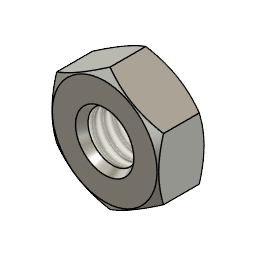
Mounting Plate (Autodesk Fusion 360 archive; units mm, degrees)
design "Hexagon Regular Nut ISO 4032 - M3 Steel 6 Plain"
description: Hexagon Regular Nut ISO 4032 - M3
part number: ISO 4032 - M3 Steel 6 Plain
Autodesk Fusion 360 part; units mm, degrees
sketch "Sketch1" plane through (0, 0, 0) normal (0, 1, 0) x (1, 0, 0)
  line L0 (0, 0) -> (0, -2.4)
  line L1 (-1.5, 0) -> (-2.695, 0)
  line L2 (-2.695, 0) -> (-3.1763, -0.2778)
  line L3 (-3.1763, -0.2778) -> (-3.1763, -2.1222)
  line L4 (-3.1763, -2.1222) -> (-2.695, -2.4)
  line L5 (-2.695, -2.4) -> (-1.5, -2.4)
  line L6 (-1.5, -2.4) -> (-1.5, 0)
  dimension "d121" = 3
  dimension "d122" = 30
  dimension "d123" = 30
  dimension "d128" = 6.3525
  dimension "d172" = 5.39
  dimension "d179" = 2.4
  constraint vertical L0
  constraint coincident L0 L0.end
  constraint coincident origin L0
  constraint horizontal L1
  constraint coincident L0.start L1
  constraint coincident L0.start origin
  constraint coincident L0.end L5
  constraint vertical L1.end L4.end
  measures "d122" angle of L1 L2
  measures "d123" angle of L4 L5
  measures "d179" distance of L1 L5
revolve "Revolve1" add sketch "Sketch1" angle 360 about axis through (0, 0, 0) along (0, 0, 1)
sketch "Sketch8" plane through (0, 0, 2.4) normal (0, 0, 1) x (1, 0, 0)
  line L0 (-2.75, -1.5894) -> (-2.75, 1.5894)
  circle A0 centre (0, 0) radius 1.5
  circle A1 centre (0, 0) radius 3.1763
  dimension "d114" = 2.75
  constraint coincident L0.end A1
  constraint coincident L0.start A1
  constraint vertical L0
  measures "d114" distance of A0.centre L0
extrude "Extrude5" cut sketch "Sketch8" against normal blind 2.4 contours L0 A1 picked at (-2.8188, -0.3871)
pattern_circular "C-Pattern2" count 6 over 360 about axis through (0, 0, 1.75) along (0, 0, 1) of "Extrude5"
thread "Thread3" "ISO Metric profile 3.0 M3x0.5 M3x0.5 6H" major diameter 3.086 minor diameter 2.529 pitch 0.5 angle 60 resizes the face on face at (-1.4925, 0.1494, 1.6)
sketch "Sketch12" plane through (0, 0, 0) normal (0, 1, 0) x (1, 0, 0)
  line L0 (-1.5, 0) -> (0, 0)
  line L1 (-0.8072, -1.2) -> (-1.5, 0)
  line L2 (-1.5, -2.4) -> (0, -2.4)
  line L3 (-0.8072, -1.2) -> (-1.5, -2.4)
  line L4 (0, 0) -> (0, -2.4)
  dimension "d169" = 60
  dimension "d177" = 1.5
  dimension "d178" = 60
  constraint horizontal L0
  constraint coincident L1.start L3.start
  constraint vertical L0.start L2.start
  constraint coincident L2.end L4.end
  constraint coincident L0.end L4.start
  constraint perpendicular L2 L4
  measures "d169" angle of L2 L3
  measures "d177" distance of L0.start L4
  measures "d178" angle of L0 L1
revolve "Revolve3" cut sketch "Sketch12" angle 360 about axis through (0, 0, 1.75) along (0, 0, 1)
equation "adsk_nheig = 2.40 mm"
equation "adsk_maxdia = 6.3525 mm"
equation "adsk_nomdia = 3.00 mm"
equation "d89 = -adsk_nheig"
equation "adsk_waflat = 5.50 mm"
equation "d114 = adsk_waflat / 2"
equation "adsk_chamang1 = 30.00 deg"
equation "adsk_chamang2 = 30.00 deg"
equation "d121 = adsk_nomdia"
equation "d122 = adsk_chamang1"
equation "d123 = adsk_chamang2"
equation "d128 = adsk_maxdia"
equation "d163 = adsk_nheig"
equation "adsk_beardia = 5.39 mm"
equation "d172 = adsk_beardia"
equation "d177 = adsk_nomdia * 0.5"
equation "d179 = adsk_nheig"

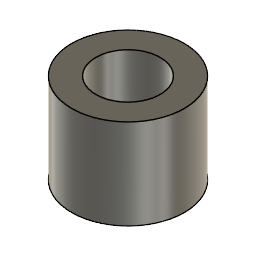
design "Standoff"
part number: 2026-01-10-15-52-55-500
Autodesk Fusion 360 part; units mm, degrees
sketch "Base" plane through (0, 0, 0) normal (0, 0, 1) x (1, 0, 0)
  circle A0 centre (0, 0) radius 5
  circle A1 centre (0, 0) radius 2.85
  circle A2 centre (0, 0) radius 2.2
  dimension "d1" = 10
  dimension "d2" = 5.7
  dimension "d3" = 4.4
  constraint coincident A0.centre A1.centre
  constraint concentric A1 A2
  measures "d1" diameter of A0
  measures "d2" diameter of A1
  measures "d3" diameter of A2
extrude "Extrude1" add sketch "Base" along normal blind 8 contours A0
extrude "Extrude2" add sketch "Base" along normal blind 2 contours A1
equation "d1 = outer_diameter"
equation "d2 = 0.95 * insert_diameter"
equation "d3 = 1.1 * inner_diameter"
equation "d4 = height"
equation "d6 = height - insert_height"
equation "outer_diameter = 10 mm"
equation "inner_diameter = 4 mm"
equation "insert_diameter = 6 mm"
equation "insert_height = 6 mm"
equation "height = 8 mm"

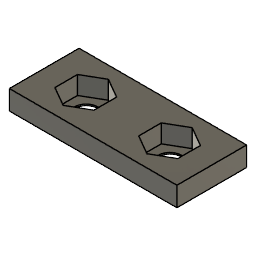
design "Bottom Connector"
part number: 2026-01-10-16-39-12-979
Autodesk Fusion 360 part; units mm, degrees
sketch "Base" plane through (0, 0, 0) normal (0, 0, 1) x (1, 0, 0)
  line L0 (12, 5) -> (-12, 5)
  line L1 (-12, 5) -> (-12, -5)
  line L2 (-12, -5) -> (12, -5)
  line L3 (12, -5) -> (12, 5)
  line L4 (12, 5) -> (-12, -5) construction
  line L5 (-12, 5) -> (12, -5) construction
  circle A0 centre (6, 0) radius 1.65
  circle A1 centre (-6, 0) radius 1.65
  dimension "d110" = 24
  dimension "d111" = 10
  dimension "d112" = 3.3
  dimension "d113" = 3.3
  constraint horizontal L0
  constraint perpendicular L0 L1
  constraint parallel L0 L2
  constraint parallel L1 L3
  constraint coincident L4 origin
  constraint coincident L5 origin
  measures "d110" distance of L1.end L2.end
  measures "d111" distance of L0.end L1.end
  measures "d112" diameter of A0
  measures "d113" diameter of A1
extrude "Extrude27" add sketch "Base" along normal blind 0.5
sketch "Nut Holders" plane through (0, 0, 0) normal (0, 0, 1) x (1, 0, 0)
  line L0 (-12, 5, 0.5) -> (12, 5, 0.5)
  line L1 (12, 5, 0.5) -> (12, -5, 0.5)
  line L2 (12, -5, 0.5) -> (-12, -5, 0.5)
  line L3 (-12, -5, 0.5) -> (-12, 5, 0.5)
  line L4 (-3.25, 1.6166, 0.5) -> (-6.05, 3.2332, 0.5)
  line L5 (-6.05, 3.2332, 0.5) -> (-8.85, 1.6166, 0.5)
  line L6 (-8.85, 1.6166, 0.5) -> (-8.85, -1.6166, 0.5)
  line L7 (-8.85, -1.6166, 0.5) -> (-6.05, -3.2332, 0.5)
  line L8 (-6.05, -3.2332, 0.5) -> (-3.25, -1.6166, 0.5)
  line L9 (-3.25, -1.6166, 0.5) -> (-3.25, 1.6166, 0.5)
  line L10 (8.75, 1.6166, 0.5) -> (5.95, 3.2332, 0.5)
  line L11 (5.95, 3.2332, 0.5) -> (3.15, 1.6166, 0.5)
  line L12 (3.15, 1.6166, 0.5) -> (3.15, -1.6166, 0.5)
  line L13 (3.15, -1.6166, 0.5) -> (5.95, -3.2332, 0.5)
  line L14 (5.95, -3.2332, 0.5) -> (8.75, -1.6166, 0.5)
  line L15 (8.75, -1.6166, 0.5) -> (8.75, 1.6166, 0.5)
  point P0 (-6.05, 0)
  point P1 (5.95, 0)
  dimension "d116" = 2.8
  dimension "d117" = 2.8
extrude "Extrude28" add sketch "Nut Holders" along normal blind 2.5 contours L0 L1 L2 L3 in plane through (0, 0, 0.5) normal (0, 0, 1)
extrude "Extrude29" cut 1 faces at (-8.45, 0, 0.5) along direction (0, 0, -1) blind 0.1
extrude "Extrude30" cut 1 faces at (3.55, 0, 0.5) along direction (0, 0, -1) blind 0.1
extrude "Extrude31" cut 1 faces at (-10.55, 0, 0) along direction (0, 0, 1) blind 0.2
move_body "Move12" bodies 1 to x (1, 0, 0) y (0, 1, 0) z (0, 0, 1) at (0, 0, -0.2)
named bodies: "Body1"

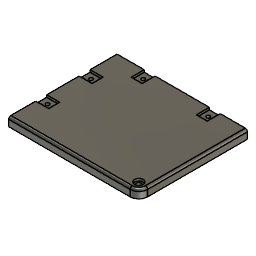
design "Corner"
part number: 2026-01-10-21-06-03-515
Autodesk Fusion 360 part; units mm, degrees
sketch "Base" plane through (0, 0, 0) normal (0, 0, 1) x (1, 0, 0)
  line L0 (60, 50) -> (-60, 50)
  line L1 (-60, 50) -> (-60, -50)
  line L2 (-60, -50) -> (60, -50)
  line L3 (60, -50) -> (60, 50)
  line L4 (60, 50) -> (-60, -50) construction
  line L5 (-60, 50) -> (60, -50) construction
  dimension "d48" = 120
  dimension "d49" = 100
  constraint horizontal L0
  constraint perpendicular L0 L1
  constraint parallel L0 L2
  constraint parallel L1 L3
  constraint coincident L4 origin
  constraint coincident L5 origin
  measures "d48" distance of L1.end L2.end
  measures "d49" distance of L0.end L1.end
extrude "Extrude16" add sketch "Base" along normal blind 8
fillet "Fillet5" radius 8 1 edges at (60, -50, 4)
fillet "Fillet6" radius 2 3 edges at (-4, -50, 8) (57.6569, -47.6569, 8) (60, 4, 8)
sketch "Top" plane through (0, 0, 8) normal (0, 0, 1) x (-1, 0, 0)
  line L0 (-58, 42) -> (-58, -50)
  line L1 (-58, -50) -> (60, -50)
  line L2 (60, -50) -> (60, 48)
  line L3 (60, 48) -> (-52, 48)
  arc A0 (-52, 48) -> (-58, 42) centre (-52, 42) ccw
  line L4 (35, -50) -> (25, -50)
  line L5 (25, -50) -> (25, -38)
  line L6 (25, -38) -> (35, -38)
  line L7 (35, -38) -> (35, -50)
  line L8 (-35, -50) -> (-25, -50)
  line L9 (-25, -50) -> (-25, -38)
  line L10 (-25, -38) -> (-35, -38)
  line L11 (-35, -38) -> (-35, -50)
  line L12 (60, -25) -> (48, -25)
  line L13 (48, -25) -> (48, -15)
  line L14 (48, -15) -> (60, -15)
  line L15 (60, -15) -> (60, -25)
  line L16 (60, 25) -> (48, 25)
  line L17 (48, 25) -> (48, 15)
  line L18 (48, 15) -> (60, 15)
  line L19 (60, 15) -> (60, 25)
  circle A1 centre (-30, -44) radius 1.65
  circle A2 centre (30, -44) radius 1.65
  circle A3 centre (54, -20) radius 1.65
  circle A4 centre (54, 20) radius 1.65
  circle A5 centre (-52, 42) radius 4
  circle A6 centre (-52, 42) radius 2.2
  dimension "d56" = 3.3
  dimension "d57" = 3.3
  dimension "d58" = 3.3
  dimension "d59" = 3.3
  dimension "d60" = 8
  dimension "d61" = 4.4
  constraint horizontal L4
  constraint vertical L5
  constraint horizontal L6
  constraint vertical L7
  constraint coincident L1 L4.start
  constraint horizontal L8
  constraint vertical L9
  constraint horizontal L10
  constraint vertical L11
  constraint coincident L1 L8.start
  constraint horizontal L12
  constraint vertical L13
  constraint horizontal L14
  constraint vertical L15
  constraint coincident L2 L12.start
  constraint horizontal L16
  constraint vertical L17
  constraint horizontal L18
  constraint vertical L19
  constraint coincident L2 L16.start
  constraint concentric A0 A5
  constraint concentric A5 A6
  measures "d56" diameter of A1
  measures "d57" diameter of A2
  measures "d58" diameter of A3
  measures "d59" diameter of A4
  measures "d60" diameter of A5
  measures "d61" diameter of A6
extrude "Extrude17" cut sketch "Top" against normal blind 2 contours A5
extrude "Extrude18" cut 1 faces at (52.3119, -40.2986, 8) along direction (0, 0, -1) through all
extrude "Extrude19" cut sketch "Top" against normal blind 2 contours L1 L8 L9 L10 L11 | L2 L16 L17 L18 L19 | L1 L4 L5 L6 L7 | L2 L12 L13 L14 L15
extrude "Extrude20" cut sketch "Top" against normal through all contours A1 | A2 | A3 | A4
sketch "Bottom" plane through (0, 0, 0) normal (0, 0, -1) x (1, 0, 0)
  circle A0 centre (-30, -44) radius 1.65
  circle A1 centre (-54, -20) radius 1.65
  circle A2 centre (30, -44) radius 1.65
  circle A3 centre (-54, 20) radius 1.65
  circle A4 centre (52, 42) radius 2.2
  arc A5 (60, 42) -> (52, 50) centre (52, 42) ccw
  line L0 (52, 50) -> (-60, 50)
  line L1 (-60, 50) -> (-60, -50)
  line L2 (-60, -50) -> (60, -50)
  line L3 (60, -50) -> (60, 42)
  line L4 (35, -50) -> (25, -50)
  line L5 (25, -50) -> (25, -38)
  line L6 (25, -38) -> (35, -38)
  line L7 (35, -38) -> (35, -50)
  line L8 (-25, -50) -> (-35, -50)
  line L9 (-35, -50) -> (-35, -38)
  line L10 (-35, -38) -> (-25, -38)
  line L11 (-25, -38) -> (-25, -50)
  line L12 (-60, -25) -> (-48, -25)
  line L13 (-48, -25) -> (-48, -15)
  line L14 (-48, -15) -> (-60, -15)
  line L15 (-60, -15) -> (-60, -25)
  line L16 (-60, 15) -> (-48, 15)
  line L17 (-48, 15) -> (-48, 25)
  line L18 (-48, 25) -> (-60, 25)
  line L19 (-60, 25) -> (-60, 15)
  constraint horizontal L4
  constraint vertical L5
  constraint horizontal L6
  constraint vertical L7
  constraint coincident L2 L4.start
  constraint horizontal L8
  constraint vertical L9
  constraint horizontal L10
  constraint vertical L11
  constraint coincident L2 L8.start
  constraint horizontal L12
  constraint vertical L13
  constraint horizontal L14
  constraint vertical L15
  constraint coincident L1 L12.start
  constraint horizontal L16
  constraint vertical L17
  constraint horizontal L18
  constraint vertical L19
  constraint coincident L1 L16.start
extrude "Extrude21" cut sketch "Bottom" against normal blind 3 contours L2 L4 L5 L6 L7 | L1 L16 L17 L18 L19 | L2 L8 L9 L10 L11 | L1 L12 L13 L14 L15
named bodies: "Body1"
